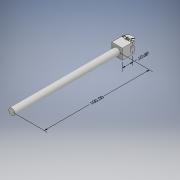
# Autodesk Inventor part: Tige
Saved by Autodesk Inventor 2018 (Build 220112000, 112)
## iProperties
Created: 2018-03-30
Part Number: Tige
Material: Générique
Document SubType Name: Modeling
Designer: Guadalix
Density: 1 g/cm^3
Appearance: Par défaut
Author: Guadalix
Autodesk Inventor part; units mm, degrees
ref_plane "YZ Plane" through (0, 0, 0) normal (1, 0, 0) x (0, 1, 0)
ref_plane "XZ Plane" through (0, 0, 0) normal (0, 1, 0) x (-1, 0, 0)
ref_plane "XY Plane" through (0, 0, 0) normal (0, 0, 1) x (1, 0, 0)
sketch "Esquisse1" plane through (0, 0, 0) normal (0, 0, 1) x (1, 0, 0)
  line L0 (-5, -5) -> (5, -5)
  line L1 (5, -5) -> (5, 5)
  line L2 (5, 5) -> (-5, 5)
  line L3 (-5, 5) -> (-5, -5)
  line L4 (-5, -5) -> (5, 5) construction
  line L5 (5, -5) -> (-5, 5) construction
  arc A0 (5, 5) -> (-5, 5) centre (0, 5) ccw
  point P0 (0, 0)
  dimension "d0" = 10
  dimension "d1" = 10
  constraints: 12 end point, 2 midpoint, 2 parallel, 2 point on circle, 1 centre point, 1 horizontal, 1 perpendicular, 1 tangent
  measures "d0" distance of L1.end L2.end
  measures "d1" distance of L0.end L1.end
extrude "Extrusion1" add sketch "Esquisse1" along normal blind 10
hole "Perçage1" at (0, 5, 10) direction (0, 0, -1) diameter 3 end through all
sketch "Esquisse3" plane through (0, 0, 0) normal (1, 0, 0) x (0, 1, 0)
  line L0 (15, 0) -> (15, 10)
  line L1 (3, 0) -> (3, 10)
  line L2 (15, 2.5) -> (3, 2.5)
  line L3 (3, 2.5) -> (3, 7.5)
  line L4 (3, 7.5) -> (15, 7.5)
  line L5 (15, 7.5) -> (15, 2.5)
  line L6 (15, 10) -> (3, 10)
  line L7 (15, 0) -> (3, 0)
  point P0 (0, 0)
  dimension "d1" = 10
  dimension "d23" = 12
  dimension "d29" = 5
  dimension "d30" = 2.5
  constraints: 16 end point, 2 parallel, 2 point on line, 1 horizontal, 1 perpendicular, 1 vertical, 2 other
  measures "d23" distance of L3.end L4.end
  measures "d29" distance between parallel lines of L2 L4
  measures "d30" distance of L4.end L0.end
extrude "Extrusion3" cut sketch "Esquisse3" along normal mid plane 100 contours L2 L1 L4 L0
sketch "Esquisse4" plane through (-5, -5, 0) normal (0, -1, 0) x (1, 0, 0)
  circle A0 centre (5, 5) radius 3
  line L0 (10, 0) -> (10, 10) projected
  line L1 (0, 10) -> (10, 10) projected
  point P0 (5, 0)
  dimension "d24" = 6
  dimension "d25" = 5
  dimension "d26" = 5
  constraints: 1 centre point
  measures "d24" diameter of A0
  measures "d25" distance from line of L0 A0.centre
  measures "d26" distance from line of L1 A0.centre
extrude "Extrusion4" add sketch "Esquisse4" along normal blind 100
